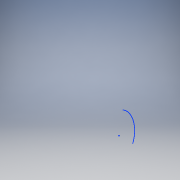
# Autodesk Inventor part: Pipe0
Saved by Autodesk Inventor 2018 (Build 220112000, 112)
## iProperties
Created: 2019-07-26
Part Number: Pipe0
Material: Generic
Document SubType Name: Modeling
Designer: micha
Density: 1 g/cm^3
Appearance: Default
Author: micha
Autodesk Inventor part; units mm, degrees
ref_plane "YZ Plane" through (0, 0, 0) normal (1, 0, 0) x (0, 1, 0)
ref_plane "XZ Plane" through (0, 0, 0) normal (0, 1, 0) x (-1, 0, 0)
ref_plane "Work Plane1" through (339.6638, 29.7399, 510.1363) normal (0.5935, 0.5795, -0.5586) x (0.8017, -0.3644, 0.4737)
sketch "Sketch1" plane through (339.6638, 29.7399, 510.1363) normal (0.5935, 0.5795, -0.5586) x (0.8017, -0.3644, 0.4737)
  arc A0 (0, 0) -> (43.6121, 0.0184) centre (21.7928, 31.32) ccw
  point P0 (-503.1541, 344.9031)
  constraints: 2 point on circle, 1 centre point
ref_plane "Work Plane2" through (339.6638, 29.7399, 510.1363) normal (0, 0, 1) x (1, 0, 0)
sketch "Sketch2" plane through (339.6638, 29.7399, 510.1363) normal (0, 0, 1) x (1, 0, 0)
  circle A0 centre (0, 0) radius 3.175
  point P0 (-339.6638, -29.7399)
  dimension "d0" = 6.35
  constraints: 1 centre point
  measures "d0" diameter of A0
sweep "Sweep1" add profiles "Sketch2" path "Sketch1"
ref_plane "Work Plane3" through (238.0638, -135.3601, 829.2238) normal (0, 1, 0) x (-1, 0, 0)
sketch "Sketch3" plane through (238.0638, -135.3601, 829.2238) normal (0, 1, 0) x (-1, 0, 0)
  ellipse E0 centre (-136.5662, -298.439) end of major axis (-133.8364, -296.8176) minor radius 2.4386 projected
  point P0 (238.0638, -829.2238)
  point P1 (-138.3976, -300.8522)
  constraints: 1 coincident, 1 other
ref_plane "Work Plane5" through (374.6299, -135.3601, 530.7847) normal (-1, 0, 0) x (0, -1, 0)
ref_plane "Work Plane4" through (390.4638, -33.7601, 524.4238) normal (-1, 0, 0) x (0, -1, 0)
sketch "Sketch4" plane through (374.6299, -135.3601, 530.7847) normal (-1, 0, 0) x (0, -1, 0)
  ellipse E0 centre (-149.1934, 0) end of major axis (-147.3437, -2.5805) minor radius 1.0383 projected
  line L0 (-149.1934, 0) -> (0.032, 0)
  point P0 (-135.3601, -530.7847)
  point P1 (-148.2433, -2.4132)
  constraints: 2 end point, 1 horizontal, 1 other
sketch "Sketch5" plane through (238.0638, -135.3601, 829.2238) normal (0, 1, 0) x (-1, 0, 0)
  circle A0 centre (-136.5873, -298.4534) radius 3.175
  point P0 (238.0638, -829.2238)
  dimension "d3" = 6.35
  constraints: 1 centre point
  measures "d3" diameter of A0
sweep "Sweep2" add profiles "Sketch3" path "Sketch4" path curves L0
body "Solid1"
